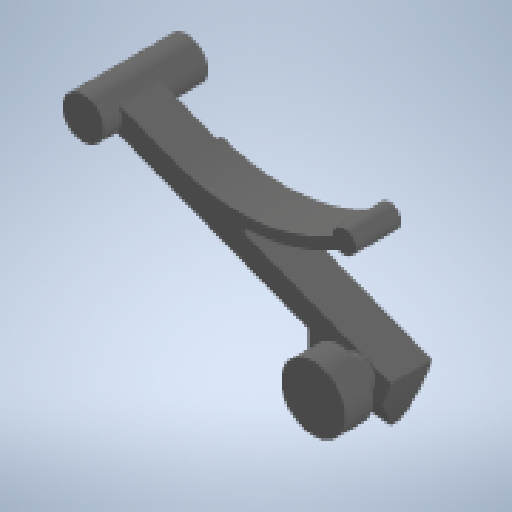
# Autodesk Inventor part: battery_holder_spring
Saved by Autodesk Inventor 2024.1 (Build 281209000, 209)
## iProperties
Created: 2025-03-30
Part Number: battery_holder_spring
Material: 一般
Document SubType Name: Modeling
Designer: hibik
Density: 1 g/cm^3
Appearance: 既定
Author: hibik
Autodesk Inventor part; units mm, degrees
ref_plane "YZ Plane" through (0, 0, 0) normal (1, 0, 0) x (0, 1, 0)
ref_plane "XZ Plane" through (0, 0, 0) normal (0, 1, 0) x (-1, 0, 0)
ref_plane "XY Plane" through (0, 0, 0) normal (0, 0, 1) x (1, 0, 0)
sketch "スケッチ1" plane through (0, 0, 0) normal (0, 0, 1) x (1, 0, 0)
  arc A0 (30.4683, -12.676) -> (31.3718, -10.2377) centre (0, 0) ccw
  circle A1 centre (0, 0) radius 2.25
  line L0 (-0.2893, -0.7459) -> (0.6509, 1.6782)
  line L1 (0.6509, 1.6782) -> (31.3718, -10.2377)
  line L2 (31.3718, -10.2377) -> (30.4316, -12.6617)
  line L3 (30.4316, -12.6617) -> (-0.2893, -0.7459)
  line L4 (-8.9792, 0) -> (38.125, 0) projected
  line L5 (30.4316, -9.873) -> (22.4316, -9.873)
  line L6 (22.4316, -9.873) -> (22.4316, -17.6617)
  line L7 (22.4316, -17.6617) -> (30.4316, -17.6617)
  line L8 (30.4316, -17.6617) -> (30.4316, -9.873)
  line L9 (22.4316, -9.873) -> (22.4316, -9.5587)
  arc A2 (30.4316, -12.764) -> (30.4683, -12.676) centre (0, 0) ccw
  point P0 (1.9096, 1.19)
  point P1 (1.6714, -1.5063)
  dimension "d0" = 33
  dimension "d1" = 4.5
  dimension "d2" = 1.8
  dimension "d4" = 0.8
  dimension "d5" = 21.2
  dimension "d6" = 8
  dimension "d7" = 5
  constraints: 18 end point, 9 point on line, 5 point on circle, 4 parallel, 3 centre point, 2 coincident, 2 concentric, 2 perpendicular, 1 horizontal
  measures "d0" radius of A0
  measures "d1" diameter of A1
  measures "d2" distance from line of L1 point (0, 0)
  measures "d4" distance from line of point (0, 0) L3
  measures "d5" angle of L4 L1
  measures "d6" distance of L6.end L7.end
  measures "d7" distance from line of L7 L2.end
extrude "押し出し1" add sketch "スケッチ1" along normal blind 4.5
sketch "スケッチ2" plane through (0, 0, 0) normal (0, 0, -1) x (-1, 0, 0)
  arc A0 (-1.6714, -1.5063) -> (-1.9096, 1.19) centre (0, 0) ccw projected
  circle A1 centre (0, 0) radius 2.25
  arc A2 (-1.6714, -1.5063) -> (-1.9096, 1.19) centre (0, 0) ccw projected
  point P0 (-1.9096, 1.19)
  point P1 (-1.6714, -1.5063)
  constraints: 1 centre point, 1 coincident, 1 concentric
extrude "押し出し2" add sketch "スケッチ2" along normal blind 4.8
sketch "スケッチ4" plane through (30.4316, -17.6617, 0) normal (1, 0, 0) x (0, 0, -1)
  line L0 (-4.5, 8.103) -> (-4.5, 0) projected
  line L1 (0, 8.103) -> (0, 0) projected
  line L2 (-4.5, 4.8977) -> (-1, 0)
  line L3 (0, 0) -> (-4.5, 0) projected
  point P0 (0, 17.6617)
  dimension "d29" = 1
  constraints: 2 end point, 1 point on line
  measures "d29" distance from line of L1 L2.end
extrude "押し出し4" cut sketch "スケッチ4" against normal through all
sketch "スケッチ5" plane through (0, 0, 4.5) normal (0, 0, 1) x (1, 0, 0)
  line L0 (1.35, 1.8) -> (36.5962, 1.8)
  arc A0 (1.9096, 1.19) -> (1.6714, -1.5063) centre (0, 0) ccw projected
  line L1 (31.3718, -10.2377) -> (1.9096, 1.19) projected
  arc A1 (8, -1.1723) -> (27, 1.8) centre (14.7895, 17.64) ccw
  arc A2 (14.1294, -3.5498) -> (28.8798, 1.8) centre (14.7895, 17.64) ccw
  circle A3 centre (26.2914, 0.55) radius 1.25
  line L2 (14.7895, 17.64) -> (26.6264, 0.0522)
  line L3 (25.9564, 1.0478) -> (14.7895, 17.64)
  line L4 (25.9564, 1.0478) -> (26.6264, 0.0522)
  point P0 (25.044, 0.4689)
  point P1 (25.6875, -0.5445)
  point P2 (27.5327, 0.6974)
  dimension "d17" = 1.8
  dimension "d18" = 1.2
  dimension "d19" = 8
  dimension "d20" = 27
  dimension "d21" = 20
  dimension "d22" = 2.5
  constraints: 8 end point, 7 point on circle, 6 point on line, 3 centre point, 2 collinear, 1 concentric, 1 horizontal, 1 midpoint, 1 tangent
  measures "d17" distance from line of L0 point (0, 0)
  measures "d18" radial gap between concentric circles of A2 A1
  measures "d19" horizontal distance of point (0, 0) A1.start
  measures "d20" horizontal distance of point (0, 0) A1.end
  measures "d21" radius of A1
  measures "d22" diameter of A3
extrude "押し出し5" add sketch "スケッチ5" against normal blind 5 contours A3 A1 L2 | A3 A2 L2 A1 | A3 A2 | L2 A1 A3 | L2 A2 A3 A1 | A3 A2 L1 A1
sketch "スケッチ6" plane through (0, 0, 4.5) normal (0, 0, 1) x (1, 0, 0)
  line L0 (22.4316, -12.764) -> (30.4316, -12.764) projected
  arc A0 (27.8759, -17.6617) -> (30.4316, -12.764) centre (0, 0) ccw
  arc A1 (30.4316, -12.764) -> (31.3718, -10.2377) centre (0, 0) ccw projected
  line L1 (22.4316, -17.6617) -> (30.4316, -17.6617) projected
  line L2 (22.4316, -17.6617) -> (22.4316, -12.764) projected
  line L3 (30.4316, -12.764) -> (30.4316, -17.6617) projected
  line L4 (22.4316, -12.764) -> (30.4316, -12.764) projected
  line L5 (30.4316, -17.6617) -> (22.4316, -17.6617) projected
  point P0 (0, 0)
  point P1 (30.4316, -12.764)
  constraints: 2 concentric, 2 point on circle, 1 centre point, 1 point on line
extrude "押し出し6" cut sketch "スケッチ6" against normal through all contours L3 L1 A0
sketch "スケッチ7" plane through (0, 0, 4.5) normal (0, 0, 1) x (1, 0, 0)
  line L0 (27.8759, -17.6617) -> (22.4316, -15.55)
  line L1 (22.4316, -17.6617) -> (22.4316, -12.764) projected
  line L2 (1.6714, -1.5063) -> (22.4316, -9.5587) projected
  arc A0 (27.8759, -17.6617) -> (30.4316, -12.764) centre (0, 0) ccw
  line L3 (22.4316, -12.764) -> (30.4316, -12.764) projected
  line L4 (22.4316, -17.6617) -> (22.4316, -12.764) projected
  line L5 (27.8759, -17.6617) -> (22.4316, -17.6617) projected
  arc A1 (30.4316, -12.764) -> (31.3718, -10.2377) centre (0, 0) ccw projected
  point P0 (0, 0)
  constraints: 2 end point, 2 point on circle, 1 centre point, 1 concentric, 1 parallel, 1 point on line
extrude "押し出し7" cut sketch "スケッチ7" against normal through all contours L5 L1 L0
sketch "スケッチ8" plane through (0, 0, 4.5) normal (0, 0, 1) x (1, 0, 0)
  line L0 (22.4316, -12.764) -> (30.4316, -12.764) projected
  arc A0 (30.4316, -12.764) -> (31.3718, -10.2377) centre (0, 0) ccw projected
  line L1 (31.3718, -10.2377) -> (14.1294, -3.5498) projected
  arc A1 (14.1294, -3.5498) -> (25.6875, -0.5445) centre (14.7895, 17.64) ccw projected
  arc A2 (25.6875, -0.5445) -> (25.044, 0.4689) centre (26.2914, 0.55) ccw projected
  arc A3 (8, -1.1723) -> (25.044, 0.4689) centre (14.7895, 17.64) ccw projected
  line L2 (8, -1.1723) -> (1.9096, 1.19) projected
  arc A4 (1.9096, 1.19) -> (1.6714, -1.5063) centre (0, 0) ccw projected
  line L3 (1.6714, -1.5063) -> (22.4316, -9.5587) projected
  line L4 (22.4316, -9.5587) -> (22.4316, -12.764) projected
  line L5 (0, 0) -> (27.9697, -10.8487)
  line L6 (27.9697, -10.8487) -> (27.5561, -11.915)
  line L7 (1.6714, -1.5063) -> (22.4316, -9.5587) projected
  circle A5 centre (27.9697, -10.8487) radius 1.8
  dimension "d34" = 30
  dimension "d35" = 3.6
  constraints: 4 end point, 1 centre point, 1 coincident, 1 parallel, 1 perpendicular
  measures "d34" distance from line of A0.centre L6
  measures "d35" diameter of A5
extrude "押し出し8" add sketch "スケッチ8" along normal blind 2 contours A5
sketch "スケッチ10" plane through (27.9697, -10.8487, 6.5) normal (0, 0, 1) x (1, 0, 0)
  circle A0 centre (0, 0) radius 1.8 projected
  circle A1 centre (0, 0) radius 3.5
  point P0 (-27.9697, 10.8487)
  dimension "d36" = 7
  constraints: 1 centre point, 1 coincident
  measures "d36" diameter of A1
extrude "押し出し10" add sketch "スケッチ10" along normal blind 3 contours A0 | A1
sketch "スケッチ11" plane through (0, 0, 4.5) normal (0, 0, 1) x (1, 0, 0)
  arc A0 (1.9096, 1.19) -> (1.6714, -1.5063) centre (0, 0) ccw projected
  circle A1 centre (0, 0) radius 2.25
  point P0 (1.6714, -1.5063)
  point P1 (1.9096, 1.19)
  constraints: 1 centre point, 1 coincident, 1 concentric
extrude "押し出し11" add sketch "スケッチ11" along normal blind 2
fillet "フィレット1" radius 0.3 1 edges at (14.1294, -3.5498, 2.25)
sketch "スケッチ12" plane through (0, 0, 0) normal (0, 0, -1) x (-1, 0, 0)
  circle A0 centre (-27.9697, -10.8487) radius 1.8 projected
  circle A1 centre (-27.9697, -10.8487) radius 1.3
  circle A2 centre (-27.9697, -10.8487) radius 0.9
  circle A3 centre (-27.9697, -10.8487) radius 0.2
  point P0 (0, 0)
  dimension "d45" = 0.4
  dimension "d46" = 0.4
  dimension "d47" = 0.5
  constraints: 3 centre point, 3 coincident
  measures "d45" diameter of A3
  measures "d46" radial gap between concentric circles of A2 A1
  measures "d47" radial gap between concentric circles of A0 A1
extrude "押し出し12" cut sketch "スケッチ12" against normal blind 8 contours A1 | A3
sketch "スケッチ13" plane through (0, 0, 0) normal (0, 0, -1) x (-1, 0, 0)
  circle A0 centre (-27.9697, -10.8487) radius 1.3 projected
  point P0 (0, 0)
extrude "押し出し13" add sketch "スケッチ13" against normal blind 0.4
pattern_linear "矩形状パターン1" count 10 spacing 1 along (0, 0, 1) of "押し出し13"
equation "\"d45\" = d46"
